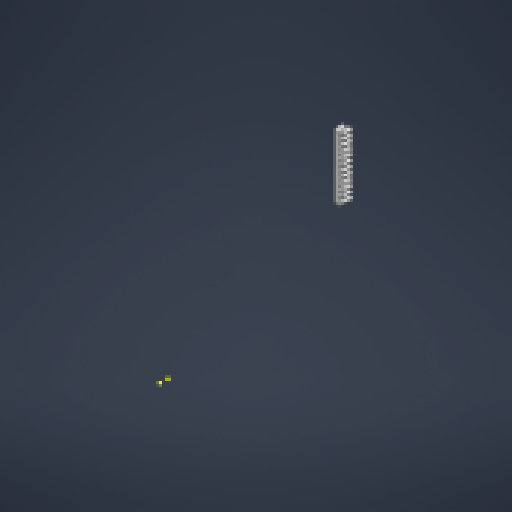
# Autodesk Inventor part: obj_2_1.齿条.STEP
Saved by Autodesk Inventor 2025 (Build 290162000, 162)
## iProperties
Created: 2026-04-25
Part Number: obj_2_1.齿条.STEP
Material: 常规
Document SubType Name: Modeling
Designer: XH
Density: 1 g/cm^3
Appearance: 默认
Author: XH
Autodesk Inventor part; units mm, degrees
ref_plane "YZ Plane" through (0, 0, 0) normal (1, 0, 0) x (0, 1, 0)
ref_plane "XZ Plane" through (0, 0, 0) normal (0, 1, 0) x (-1, 0, 0)
ref_plane "XY Plane" through (0, 0, 0) normal (0, 0, 1) x (1, 0, 0)
sketch "草图3" plane through (0, 0, 0) normal (0, 1, 0) x (-1, 0, 0)
  point P0 (0, 0)
sketch "草图4" plane through (0, 0, 0) normal (0, 0, 1) x (1, 0, 0)
  line L0 (96.7568, 180.6564) -> (96.7568, 80.6564) projected
  line L1 (99.6318, 180.6564) -> (96.7568, 180.6564) projected
  line L2 (105.5068, 180.6564) -> (102.6318, 180.6564) projected
  circle A0 centre (101.1316, 180.6563) radius 1.4998 projected
  line L3 (107.7568, 179.4984) -> (105.5068, 180.0803) projected
  line L4 (105.5068, 80.6564) -> (105.5068, 180.6564) projected
  line L5 (105.5068, 178.091) -> (107.7568, 178.6728) projected
  line L6 (107.7568, 179.4984) -> (107.7568, 178.6728) projected
  line L7 (107.7568, 176.3568) -> (107.7568, 175.5313) projected
  line L8 (107.7568, 175.5313) -> (105.5068, 174.9494) projected
  line L9 (105.5068, 176.9387) -> (107.7568, 176.3568) projected
  line L10 (105.5068, 173.7971) -> (107.7568, 173.2152) projected
  line L11 (107.7568, 173.2152) -> (107.7568, 172.3897) projected
  line L12 (107.7568, 172.3897) -> (102.5791, 171.0506) projected
  line L13 (105.5068, 170.6555) -> (107.7568, 170.0736) projected
  line L14 (107.7568, 170.0736) -> (107.7568, 169.2481) projected
  line L15 (107.7568, 169.2481) -> (105.5068, 168.6662) projected
  line L16 (105.5068, 167.5139) -> (107.7568, 166.932) projected
  line L17 (107.7568, 166.1065) -> (105.5068, 165.5246) projected
  line L18 (107.7568, 166.932) -> (107.7568, 166.1065) projected
  line L19 (105.5068, 164.3723) -> (107.7568, 163.7905) projected
  line L20 (107.7568, 163.7905) -> (107.7568, 162.9649) projected
  line L21 (107.7568, 162.9649) -> (105.5068, 162.383) projected
  line L22 (105.5068, 161.2307) -> (107.7568, 160.6488) projected
  line L23 (107.7568, 160.6488) -> (107.7568, 159.8233) projected
  line L24 (107.7568, 159.8233) -> (105.5068, 159.2414) projected
  line L25 (105.5068, 158.0892) -> (107.7568, 157.5073) projected
  line L26 (107.7568, 157.5073) -> (107.7568, 156.6817) projected
  line L27 (107.7568, 156.6817) -> (105.5068, 156.0998) projected
  line L28 (105.5068, 154.9476) -> (107.7568, 154.3657) projected
  line L29 (107.7568, 154.3657) -> (107.7568, 153.5401) projected
  line L30 (107.7568, 153.5401) -> (105.5068, 152.9582) projected
  line L31 (105.5068, 151.806) -> (107.7568, 151.2241) projected
  line L32 (107.7568, 151.2241) -> (107.7568, 150.3985) projected
  line L33 (107.7568, 150.3985) -> (105.5068, 149.8166) projected
  line L34 (105.5068, 148.6644) -> (107.7568, 148.0825) projected
  line L35 (107.7568, 148.0825) -> (107.7568, 147.2569) projected
  line L36 (107.7568, 147.2569) -> (105.5068, 146.675) projected
  line L37 (105.5068, 145.5228) -> (107.7568, 144.9409) projected
  line L38 (107.7568, 144.9409) -> (107.7568, 144.1153) projected
  line L39 (107.7568, 144.1153) -> (105.5068, 143.5334) projected
  line L40 (105.5068, 142.3812) -> (107.7568, 141.7993) projected
  line L41 (107.7568, 141.7993) -> (107.7568, 140.9737) projected
  line L42 (107.7568, 140.9737) -> (105.5068, 140.3918) projected
  line L43 (102.4905, 140.0197) -> (107.7568, 138.6577) projected
  line L44 (107.7568, 138.6577) -> (107.7568, 137.8321) projected
  line L45 (107.7568, 137.8321) -> (105.5068, 137.2503) projected
  line L46 (105.5068, 136.098) -> (107.7568, 135.5161) projected
  line L47 (107.7568, 135.5161) -> (107.7568, 134.6906) projected
  line L48 (107.7568, 134.6906) -> (105.5068, 134.1087) projected
  line L49 (105.5068, 132.9564) -> (107.7568, 132.3745) projected
  line L50 (107.7568, 132.3745) -> (107.7568, 131.549) projected
  line L51 (107.7568, 131.549) -> (105.5068, 130.9671) projected
  line L52 (105.5068, 129.8148) -> (107.7568, 129.2329) projected
  line L53 (107.7568, 129.2329) -> (107.7568, 128.4074) projected
  line L54 (107.7568, 128.4074) -> (105.5068, 127.8255) projected
  line L55 (105.5068, 126.6732) -> (107.7568, 126.0913) projected
  line L56 (107.7568, 126.0913) -> (107.7568, 125.2658) projected
  line L57 (107.7568, 125.2658) -> (105.5068, 124.6839) projected
  line L58 (105.5068, 123.5316) -> (107.7568, 122.9497) projected
  line L59 (107.7568, 122.1242) -> (102.6236, 120.7967) projected
  line L60 (107.7568, 122.9497) -> (107.7568, 122.1242) projected
  circle A1 centre (101.1329, 170.6543) radius 1.5024 projected
  circle A2 centre (101.1319, 160.6561) radius 1.5003 projected
  circle A3 centre (101.1312, 150.656) radius 1.4993 projected
  circle A4 centre (101.1297, 140.6572) radius 1.4978 projected
  circle A5 centre (101.1313, 130.6569) radius 1.4993 projected
  circle A6 centre (101.1332, 120.6547) radius 1.5023 projected
  line L61 (105.5068, 120.39) -> (107.7568, 119.8081) projected
  line L62 (107.7568, 119.8081) -> (107.7568, 118.9826) projected
  line L63 (107.7568, 118.9826) -> (105.5068, 118.4007) projected
  line L64 (105.5068, 117.2484) -> (107.7568, 116.6666) projected
  line L65 (107.7568, 116.6666) -> (107.7568, 115.841) projected
  line L66 (107.7568, 115.841) -> (105.5068, 115.2591) projected
  line L67 (105.5068, 114.1069) -> (107.7568, 113.525) projected
  line L68 (107.7568, 112.6994) -> (105.5068, 112.1175) projected
  line L69 (107.7568, 113.525) -> (107.7568, 112.6994) projected
  line L70 (105.5068, 110.9653) -> (107.7568, 110.3834) projected
  line L71 (107.7568, 110.3834) -> (107.7568, 109.5578) projected
  line L72 (107.7568, 109.5578) -> (105.5068, 108.9759) projected
  line L73 (105.5068, 104.6821) -> (107.7568, 104.1002) projected
  line L74 (107.7568, 106.4162) -> (105.5068, 105.8343) projected
  line L75 (105.5068, 107.8237) -> (107.7568, 107.2418) projected
  line L76 (107.7568, 107.2418) -> (107.7568, 106.4162) projected
  line L77 (107.7568, 104.1002) -> (107.7568, 103.2746) projected
  line L78 (107.7568, 103.2746) -> (102.0947, 101.8103) projected
  line L79 (105.5068, 101.5405) -> (107.7568, 100.9586) projected
  line L80 (107.7568, 100.9586) -> (107.7568, 100.133) projected
  line L81 (107.7568, 100.133) -> (105.5068, 99.5511) projected
  circle A7 centre (101.1318, 100.6565) radius 1.5 projected
  line L82 (105.5068, 80.6564) -> (102.6318, 80.6564) projected
  line L83 (99.6318, 80.6564) -> (96.7568, 80.6564) projected
  line L84 (96.7568, 80.6564) -> (96.7568, 180.6564) projected
  line L85 (105.5068, 92.1157) -> (107.7568, 91.5338) projected
  line L86 (107.7568, 91.5338) -> (107.7568, 90.7083) projected
  line L87 (107.7568, 90.7083) -> (105.5068, 90.1264) projected
  line L88 (107.7568, 93.8498) -> (105.5068, 93.268) projected
  line L89 (107.7568, 94.6754) -> (107.7568, 93.8498) projected
  line L90 (105.5068, 95.2573) -> (107.7568, 94.6754) projected
  line L91 (107.7568, 96.9914) -> (105.5068, 96.4095) projected
  line L92 (105.5068, 98.3989) -> (107.7568, 97.817) projected
  line L93 (107.7568, 97.817) -> (107.7568, 96.9914) projected
  line L94 (107.7568, 88.3922) -> (107.7568, 87.5667) projected
  line L95 (102.3585, 89.7883) -> (107.7568, 88.3922) projected
  circle A8 centre (101.1321, 90.6562) radius 1.5004 projected
  line L96 (107.7568, 87.5667) -> (105.5068, 86.9848) projected
  line L97 (105.5068, 85.8325) -> (107.7568, 85.2506) projected
  line L98 (107.7568, 85.2506) -> (107.7568, 84.4251) projected
  line L99 (107.7568, 84.4251) -> (105.5068, 83.8432) projected
  line L100 (105.5068, 82.6909) -> (107.7568, 82.109) projected
  line L101 (107.7568, 82.109) -> (107.7568, 81.2835) projected
  line L102 (107.7568, 81.2835) -> (105.5068, 80.7016) projected
  circle A9 centre (101.1318, 80.6565) radius 1.5 projected
  line L103 (96.7568, 80.6564) -> (105.5068, 80.6564)
  line L104 (105.5068, 80.6564) -> (105.5068, 180.6564)
  line L105 (105.5068, 180.6564) -> (96.7568, 180.6564)
  line L106 (96.7568, 180.6564) -> (96.7568, 80.6564)
  point P0 (0, 0)
  point P1 (105.5068, 171.8078)
  point P2 (102.6314, 180.6564)
  point P3 (99.6318, 180.6564)
  point P4 (99.6318, 80.6564)
  point P5 (102.6317, 80.6564)
  point P6 (105.5068, 88.9741)
  point P7 (105.5068, 102.6927)
  point P8 (105.5068, 121.5423)
  point P9 (105.5068, 139.2396)
  constraints: 8 end point, 2 parallel, 1 horizontal, 1 perpendicular, 1 other
extrude "拉伸2" add sketch "草图4" along normal blind 4 contours L1 A0 L2 L4 L82 A9 L83 L0 | L3 L6 L5 L4 | L4 L100 L101 L102 | L9 L7 L8 L4 | L4 L97 L98 L99 | L10 L11 L12 L4 | L4 L95 L94 L96 | L13 L14 L15 L4 | L4 L85 L86 L87 | L16 L18 L17 L4 | L4 L90 L89 L88 | L19 L20 L21 L4 | L4 L92 L93 L91 | L22 L23 L24 L4 | L4 L79 L80 L81 | L25 L26 L27 L4 | L4 L73 L77 L78 | L28 L29 L30 L4 | L4 L75 L76 L74 | L31 L32 L33 L4 | L4 L70 L71 L72 | L34 L35 L36 L4 | L4 L67 L69 L68 | L37 L38 L39 L4 | L4 L64 L65 L66 | L40 L41 L42 L4 | L4 L61 L62 L63 | L43 L44 L45 L4 | L4 L58 L60 L59 | L46 L47 L48 L4 | L4 L55 L56 L57 | L49 L50 L51 L4 | L4 L52 L53 L54
sketch "草图5" plane through (0, 0, 0) normal (0, 0, -1) x (-1, 0, 0)
  line L0 (-88.0523, 73.2869) -> (-124.347, 73.2869)
  line L1 (-124.347, 73.2869) -> (-124.347, 102.0841)
  line L2 (-124.347, 102.0841) -> (-88.0523, 102.0841)
  line L3 (-88.0523, 102.0841) -> (-88.0523, 73.2869)
  line L4 (-119.7058, 102.0841) -> (-61.5255, 102.0841) projected
  point P0 (0, 0)
  constraints: 8 end point, 2 parallel, 1 collinear, 1 horizontal, 1 perpendicular
extrude "拉伸3" cut sketch "草图5" against normal blind 4
delete faces "删除1" heal yes whole lump no faces at (101.4922, 102.1125, 2.6667)
delete faces "删除2" heal yes whole lump no faces at (101.0714, 179.1577, 2.6667)
delete faces "删除3" heal yes whole lump no faces at (102.558, 170.1785, 2.6667) (102.6274, 160.5354, 2.6667) (102.0794, 151.8173, 2.6667) (102.5077, 141.2443, 2.6667) (102.5535, 130.1821, 2.6667) (101.0727, 122.1557, 2.6667)
sketch "草图9" plane through (96.7568, 180.6564, 4) normal (0, 0, 1) x (1, 0, 0)
  point P0 (-96.7568, -180.6564)
sketch "草图10" plane through (96.7568, 180.6564, 4) normal (0, 0, 1) x (1, 0, 0)
  line L0 (8.75, 0) -> (0, 0) projected
  line L1 (5, 0) -> (11, 0)
  line L2 (11, 0) -> (11, -78.5724)
  line L3 (11, -78.5724) -> (5, -78.5724)
  line L4 (5, -78.5724) -> (5, 0)
  line L5 (11, -77.3818) -> (11, -76.5562) projected
  line L6 (0, -78.5724) -> (8.75, -78.5724) projected
  line L7 (8.75, 0) -> (0, 0) projected
  line L8 (0, 0) -> (0, -78.5724) projected
  line L9 (0, -78.5724) -> (8.75, -78.5724) projected
  line L10 (8.75, -78.5724) -> (8.75, -77.9637) projected
  line L11 (8.75, -77.9637) -> (11, -77.3818) projected
  line L12 (11, -77.3818) -> (11, -76.5562) projected
  line L13 (11, -76.5562) -> (8.75, -75.9744) projected
  line L14 (8.75, -75.9744) -> (8.75, -74.8221) projected
  line L15 (8.75, -74.8221) -> (11, -74.2402) projected
  line L16 (11, -74.2402) -> (11, -73.4147) projected
  line L17 (11, -73.4147) -> (8.75, -72.8328) projected
  line L18 (8.75, -72.8328) -> (8.75, -71.6805) projected
  line L19 (8.75, -71.6805) -> (11, -71.0986) projected
  line L20 (11, -71.0986) -> (11, -70.2731) projected
  line L21 (11, -70.2731) -> (8.75, -69.6912) projected
  line L22 (8.75, -69.6912) -> (8.75, -68.5389) projected
  line L23 (8.75, -68.5389) -> (11, -67.957) projected
  line L24 (11, -67.957) -> (11, -67.1315) projected
  line L25 (11, -67.1315) -> (8.75, -66.5496) projected
  line L26 (8.75, -66.5496) -> (8.75, -65.3973) projected
  line L27 (8.75, -65.3973) -> (11, -64.8154) projected
  line L28 (11, -64.8154) -> (11, -63.9899) projected
  line L29 (11, -63.9899) -> (8.75, -63.408) projected
  line L30 (8.75, -63.408) -> (8.75, -62.2557) projected
  line L31 (8.75, -62.2557) -> (11, -61.6738) projected
  line L32 (11, -61.6738) -> (11, -60.8483) projected
  line L33 (11, -60.8483) -> (8.75, -60.2664) projected
  line L34 (8.75, -60.2664) -> (8.75, -59.1141) projected
  line L35 (8.75, -59.1141) -> (11, -58.5322) projected
  line L36 (11, -58.5322) -> (11, -57.7067) projected
  line L37 (11, -57.7067) -> (8.75, -57.1248) projected
  line L38 (8.75, -57.1248) -> (8.75, -55.9725) projected
  line L39 (8.75, -55.9725) -> (11, -55.3907) projected
  line L40 (11, -55.3907) -> (11, -54.5651) projected
  line L41 (11, -54.5651) -> (8.75, -53.9832) projected
  line L42 (8.75, -53.9832) -> (8.75, -52.831) projected
  line L43 (8.75, -52.831) -> (11, -52.2491) projected
  line L44 (11, -52.2491) -> (11, -51.4235) projected
  line L45 (11, -51.4235) -> (8.75, -50.8416) projected
  line L46 (8.75, -50.8416) -> (8.75, -49.6894) projected
  line L47 (8.75, -49.6894) -> (11, -49.1075) projected
  line L48 (11, -49.1075) -> (11, -48.2819) projected
  line L49 (11, -48.2819) -> (8.75, -47.7) projected
  line L50 (8.75, -47.7) -> (8.75, -46.5478) projected
  line L51 (8.75, -46.5478) -> (11, -45.9659) projected
  line L52 (11, -45.9659) -> (11, -45.1403) projected
  line L53 (11, -45.1403) -> (8.75, -44.5584) projected
  line L54 (8.75, -44.5584) -> (8.75, -43.4062) projected
  line L55 (8.75, -43.4062) -> (11, -42.8243) projected
  line L56 (11, -42.8243) -> (11, -41.9987) projected
  line L57 (11, -41.9987) -> (8.75, -41.4168) projected
  line L58 (8.75, -41.4168) -> (8.75, -40.2646) projected
  line L59 (8.75, -40.2646) -> (11, -39.6827) projected
  line L60 (11, -39.6827) -> (11, -38.8571) projected
  line L61 (11, -38.8571) -> (8.75, -38.2752) projected
  line L62 (8.75, -38.2752) -> (8.75, -37.123) projected
  line L63 (8.75, -37.123) -> (11, -36.5411) projected
  line L64 (11, -36.5411) -> (11, -35.7155) projected
  line L65 (11, -35.7155) -> (8.75, -35.1336) projected
  line L66 (8.75, -35.1336) -> (8.75, -33.9814) projected
  line L67 (8.75, -33.9814) -> (11, -33.3995) projected
  line L68 (11, -33.3995) -> (11, -32.5739) projected
  line L69 (11, -32.5739) -> (8.75, -31.9921) projected
  line L70 (8.75, -31.9921) -> (8.75, -30.8398) projected
  line L71 (8.75, -30.8398) -> (11, -30.2579) projected
  line L72 (11, -30.2579) -> (11, -29.4324) projected
  line L73 (11, -29.4324) -> (8.75, -28.8505) projected
  line L74 (8.75, -28.8505) -> (8.75, -27.6982) projected
  line L75 (8.75, -27.6982) -> (11, -27.1163) projected
  line L76 (11, -27.1163) -> (11, -26.2908) projected
  line L77 (11, -26.2908) -> (8.75, -25.7089) projected
  line L78 (8.75, -25.7089) -> (8.75, -24.5566) projected
  line L79 (8.75, -24.5566) -> (11, -23.9747) projected
  line L80 (11, -23.9747) -> (11, -23.1492) projected
  line L81 (11, -23.1492) -> (8.75, -22.5673) projected
  line L82 (8.75, -22.5673) -> (8.75, -21.415) projected
  line L83 (8.75, -21.415) -> (11, -20.8331) projected
  line L84 (11, -20.8331) -> (11, -20.0076) projected
  line L85 (11, -20.0076) -> (8.75, -19.4257) projected
  line L86 (8.75, -19.4257) -> (8.75, -18.2734) projected
  line L87 (8.75, -18.2734) -> (11, -17.6915) projected
  line L88 (11, -17.6915) -> (11, -16.866) projected
  line L89 (11, -16.866) -> (8.75, -16.2841) projected
  line L90 (8.75, -16.2841) -> (8.75, -15.1319) projected
  line L91 (8.75, -15.1319) -> (11, -14.55) projected
  line L92 (11, -14.55) -> (11, -13.7244) projected
  line L93 (11, -13.7244) -> (8.75, -13.1425) projected
  line L94 (8.75, -13.1425) -> (8.75, -11.9902) projected
  line L95 (8.75, -11.9902) -> (11, -11.4083) projected
  line L96 (11, -11.4083) -> (11, -10.5828) projected
  line L97 (11, -10.5828) -> (8.75, -10.0009) projected
  line L98 (8.75, -10.0009) -> (8.75, -8.8487) projected
  line L99 (8.75, -8.8487) -> (11, -8.2668) projected
  line L100 (11, -8.2668) -> (11, -7.4412) projected
  line L101 (11, -7.4412) -> (8.75, -6.8593) projected
  line L102 (8.75, -6.8593) -> (8.75, -5.7071) projected
  line L103 (8.75, -5.7071) -> (11, -5.1252) projected
  line L104 (11, -5.1252) -> (11, -4.2996) projected
  line L105 (11, -4.2996) -> (8.75, -3.7177) projected
  line L106 (8.75, -3.7177) -> (8.75, -2.5655) projected
  line L107 (8.75, -2.5655) -> (11, -1.9836) projected
  line L108 (11, -1.9836) -> (11, -1.158) projected
  line L109 (11, -1.158) -> (8.75, -0.5761) projected
  line L110 (8.75, -0.5761) -> (8.75, 0) projected
  point P0 (-96.7568, -180.6564)
  dimension "d16" = 5
  constraints: 8 end point, 2 collinear, 2 parallel, 1 horizontal, 1 perpendicular, 1 point on line
  measures "d16" distance between parallel lines of L8 L4
extrude "拉伸6" cut sketch "草图10" against normal blind 10 contours L4 L6 L8 L0
sketch "草图11" plane through (101.7568, 102.0841, 4) normal (0, 0, 1) x (1, 0, 0)
  point P0 (-101.7568, -102.0841)
sketch "草图12" plane through (101.7568, 102.0841, 4) normal (0, 0, 1) x (1, 0, 0)
  line L0 (-1.8631, -5.8969) -> (10.9034, -5.8969)
  line L1 (10.9034, -5.8969) -> (10.9034, 40)
  line L2 (10.9034, 40) -> (-1.8631, 40)
  line L3 (-1.8631, 40) -> (-1.8631, -5.8969)
  line L4 (0, 0) -> (3.75, 0) projected
  point P0 (-101.7568, -102.0841)
  point P1 (3.5629, 40)
  point P2 (1.875, 0)
  dimension "d22" = 40
  constraints: 8 end point, 2 parallel, 1 horizontal, 1 midpoint, 1 perpendicular, 1 point on line
  measures "d22" distance from line of L2 point (1.875, 0)
extrude "拉伸7" cut sketch "草图12" against normal blind 14
sketch "草图13" plane through (105.5068, 161.2307, 4) normal (0, 0, 1) x (1, 0, 0)
  ellipse E0 centre (-1.8796, 19.353) end of major axis (-0.8191, 18.2921) minor radius 1.5 projected
  point P0 (-105.5068, -161.2307)
extrude "拉伸8" cut sketch "草图13" against normal blind 10
fillet "圆角1" radius 0.1 2 edges at (102.1289, 180.6564, 2.0021) (105.1254, 180.6564, 2.0021)
delete faces "删除4" heal yes whole lump no faces at (106.2727, 142.1831, 1.3333)
sketch "草图14" plane through (101.7568, 142.0841, 4) normal (0, 0, 1) x (1, 0, 0)
  ellipse E0 centre (1.8704, 38.4996) end of major axis (2.9309, 37.4388) minor radius 1.5 (0.3706, 38.4741) -> (3.3702, 38.4741) ccw projected
  circle A0 centre (1.8704, 38.4996) radius 2
  point P0 (-101.7568, -142.0841)
  dimension "d23" = 4
  constraints: 1 centre point, 1 coincident, 1 other
  measures "d23" diameter of A0
extrude "拉伸9" cut sketch "草图14" against normal blind 10
fillet "圆角2" radius 0.1 2 edges at (101.7568, 179.8755, 2) (105.5592, 180.0667, 2)
move faces "移动1" translate (0, 0, 1) faces at (103.0068, 159.2127, 4)
